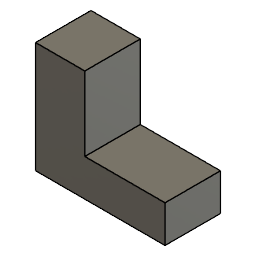
replay (Autodesk Fusion 360 design; units mm, degrees)
Autodesk Fusion 360 part; units mm, degrees
sketch "草图1" plane through (0, 0, 0) normal (0, 0, 1) x (1, 0, 0)
  line L0 (42, 0) -> (42, 12)
  line L1 (42, 12) -> (16, 12)
  line L2 (16, 12) -> (16, 36)
  line L3 (16, 36) -> (0, 36)
  line L4 (0, 36) -> (0, 0)
  line L5 (0, 0) -> (42, 0)
extrude "拉伸1" add sketch "草图1" along normal blind 18
